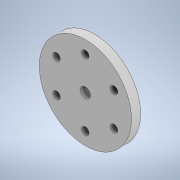
# Autodesk Inventor part: capp
Saved by Autodesk Inventor 2022 (Build 260153000, 153)
## iProperties
Created: 2022-03-10
Part Number: capp
Material: Generic
Document SubType Name: Sheet Metal
Designer: karee
Density: 1 g/cm^3
Sheet Metal Rule: Default
Appearance: Default
Author: karee
Autodesk Inventor part; units mm, degrees
ref_plane "YZ Plane" through (0, 0, 0) normal (1, 0, 0) x (0, 1, 0)
ref_plane "XZ Plane" through (0, 0, 0) normal (0, 1, 0) x (-1, 0, 0)
ref_plane "XY Plane" through (0, 0, 0) normal (0, 0, 1) x (1, 0, 0)
sketch "Sketch1" plane through (0, 0, 0) normal (0, 0, 1) x (1, 0, 0)
  point P0 (0, 0)
sketch "Sketch2" plane through (0, 0, 0) normal (0, 0, 1) x (1, 0, 0)
  circle A0 centre (0, 0) radius 50
  dimension "d0" = 100
  constraints: 1 centre point, 1 coincident
  measures "d0" diameter of A0
extrude "Extrusion1" add sketch "Sketch2" along normal blind 10
sketch "Sketch5" plane through (0, 0, 10) normal (0, 0, 1) x (1, 0, 0)
  circle A0 centre (0, 0) radius 12.5 projected
  line L0 (0, 0) -> (0, 36)
  circle A1 centre (0, 36) radius 4
  dimension "d16" = 36
  dimension "d17" = 8
  constraints: 2 end point, 1 centre point, 1 coincident, 1 vertical
  measures "d16" distance of L0.start L0.end
  measures "d17" diameter of A1
extrude "Extrusion4" cut sketch "Sketch5" against normal blind 10 contours A1
sketch "Sketch7" plane through (0, 0, 10) normal (0, 0, 1) x (1, 0, 0)
  circle A0 centre (0, 0) radius 5.5
  dimension "d26" = 11
  constraints: 1 centre point, 1 coincident
  measures "d26" diameter of A0
extrude "Extrusion6" cut sketch "Sketch7" against normal blind 10
pattern_circular "Circular Pattern2" count 6 over 360 about axis through (0, 0, 10) along (0, 0, -1) of "Extrusion4"
equation "\"BendRadius\" = Thickness"
equation "\"BendReliefWidth\" = Thickness"
equation "\"BendReliefDepth\" = 0.5 * Thickness"
equation "\"CornerReliefSize\" = 4 * Thickness"
equation "\"MinimumRemnant\" = 2 * Thickness"
equation "\"TransitionRadius\" = BendRadius"
equation "\"JacobiRadiusSize\" = BendRadius"
equation "\"GapSize\" = Thickness"
equation "\"Thickness\" = 3.048"
body "Solid1"
